Autodesk Inventor part; units mm, degrees
(part 2 of 2)
  spline S84 degree 3 poles (-140.8814, 47.3494) (-140.881, 47.3593) (-140.8802, 47.3795) (-140.879, 47.3997) (-140.8784, 47.4099) knots 0 0 0 0 0.002981 0.006062 0.006062 0.006062 0.006062 projected
  line L286 (-140.8784, 47.4099) -> (-141.648, 47.4099) projected
  spline S85 degree 3 poles (-141.648, 47.4099) (-141.7169, 47.4116) (-141.8249, 47.4142) (-141.923, 47.3709) (-141.9585, 47.3552) knots 0 0 0 0 0.02031 0.031854 0.031854 0.031854 0.031854 projected
  spline S86 degree 3 poles (-141.9585, 47.3552) (-141.9835, 47.3257) (-142.0377, 47.2619) (-142.0421, 47.1778) (-142.0445, 47.1326) knots 0 0 0 0 0.011297 0.024461 0.024461 0.024461 0.024461 projected
  line L287 (-142.0445, 47.1326) -> (-142.0445, 47.0291) projected
  line L288 (-142.0445, 47.0291) -> (-142.1167, 47.0291) projected
  line L289 (-142.1167, 47.0291) -> (-142.1167, 48.1638) projected
  line L290 (-142.1167, 48.1638) -> (-142.0445, 48.1638) projected
  line L291 (-142.0445, 48.1638) -> (-142.0445, 48.0642) projected
  spline S87 degree 3 poles (-142.0445, 48.0642) (-142.0414, 48.0133) (-142.0357, 47.9185) (-141.9669, 47.8539) (-141.9351, 47.824) knots 0 0 0 0 0.014662 0.027303 0.027303 0.027303 0.027303 projected
  spline S88 degree 3 poles (-141.9351, 47.824) (-141.9013, 47.8122) (-141.8089, 47.78) (-141.7105, 47.7818) (-141.648, 47.783) knots 0 0 0 0 0.010659 0.029193 0.029193 0.029193 0.029193 projected
  line L292 (-141.648, 47.783) -> (-139.937, 47.783) projected
  spline S89 degree 3 poles (-139.937, 47.783) (-139.8681, 47.7813) (-139.7601, 47.7787) (-139.662, 47.822) (-139.6265, 47.8377) knots 0 0 0 0 0.02031 0.031854 0.031854 0.031854 0.031854 projected
  spline S90 degree 3 poles (-139.6265, 47.8377) (-139.6015, 47.8678) (-139.5473, 47.9331) (-139.5429, 48.0184) (-139.5405, 48.0642) knots 0 0 0 0 0.011457 0.024815 0.024815 0.024815 0.024815 projected
  line L293 (-139.5405, 48.0642) -> (-139.5405, 48.1638) projected
  line L294 (-139.5405, 48.1638) -> (-139.4683, 48.1638) projected
  line L295 (-139.4683, 48.1638) -> (-139.4683, 47.199) projected
  spline S91 degree 3 poles (-139.4683, 47.199) (-139.4686, 47.0763) (-139.469, 46.8667) (-139.512, 46.6618) (-139.5298, 46.5769) knots 0 0 0 0 0.036678 0.062652 0.062652 0.062652 0.062652 projected
  spline S92 degree 3 poles (-139.5298, 46.5769) (-139.5549, 46.5125) (-139.6054, 46.3826) (-139.7058, 46.2859) (-139.7564, 46.2371) knots 0 0 0 0 0.020466 0.04128 0.04128 0.04128 0.04128 projected
  spline S93 degree 3 poles (-139.7564, 46.2371) (-139.8146, 46.1963) (-139.9328, 46.1136) (-140.0768, 46.1029) (-140.1499, 46.0974) knots 0 0 0 0 0.020904 0.042453 0.042453 0.042453 0.042453 projected
  spline S94 degree 3 poles (-140.1499, 46.0974) (-140.2285, 46.1039) (-140.3849, 46.1169) (-140.511, 46.2102) (-140.5738, 46.2566) knots 0 0 0 0 0.023147 0.04608 0.04608 0.04608 0.04608 projected
  spline S95 degree 3 poles (-140.5738, 46.2566) (-140.6301, 46.3214) (-140.7547, 46.4645) (-140.8018, 46.6489) (-140.8277, 46.7498) knots 0 0 0 0 0.02543 0.056151 0.056151 0.056151 0.056151 projected
  line L296 (-140.8277, 46.7498) -> (-141.5874, 46.2029) projected
  spline S96 degree 3 poles (-141.5874, 46.2029) (-141.6633, 46.1482) (-141.7928, 46.055) (-141.8934, 45.9317) (-141.9351, 45.8806) knots 0 0 0 0 0.027895 0.047582 0.047582 0.047582 0.047582 projected
  spline S97 degree 3 poles (-141.9351, 45.8806) (-141.9614, 45.8298) (-142.0185, 45.7192) (-142.0353, 45.5957) (-142.0445, 45.5291) knots 0 0 0 0 0.017045 0.037059 0.037059 0.037059 0.037059 projected
  line L297 (-142.0445, 45.5291) -> (-142.1167, 45.5291) projected
  circle A54 centre (-140.23, -52.19) radius 0.7 projected
  circle A55 centre (-140.23, -11.13) radius 0.7 projected
  circle A56 centre (-140.23, -6.05) radius 0.7 projected
  circle A57 centre (-140.23, -0.97) radius 0.7 projected
  circle A58 centre (-140.23, 4.11) radius 0.7 projected
  circle A59 centre (-140.23, 9.19) radius 0.7 projected
  circle A60 centre (-140.23, 11.73) radius 0.7 projected
  circle A61 centre (-140.23, 6.65) radius 0.7 projected
  circle A62 centre (-140.23, 1.57) radius 0.7 projected
  circle A63 centre (-140.23, -3.51) radius 0.7 projected
  circle A64 centre (-140.23, -8.59) radius 0.7 projected
  circle A65 centre (-140.23, -49.65) radius 0.7 projected
  circle A66 centre (-140.23, -54.73) radius 0.7 projected
  circle A67 centre (-100.1, -55.5) radius 0.7 projected
  circle A68 centre (-100.1, -45.5) radius 0.7 projected
  circle A69 centre (-100.1, -35.5) radius 0.7 projected
  circle A70 centre (-100.1, -23.5) radius 0.7 projected
  circle A71 centre (-100.1, -13.5) radius 0.7 projected
  circle A72 centre (-100.1, -3.5) radius 0.7 projected
  circle A73 centre (-100.1, 8.5) radius 0.7 projected
  circle A74 centre (-100.1, 13.5) radius 0.7 projected
  circle A75 centre (-100.1, 28.5) radius 0.7 projected
  circle A76 centre (-100.1, 40.5) radius 0.7 projected
  circle A77 centre (-100.1, 50.5) radius 0.7 projected
  circle A78 centre (-100.1, 60.5) radius 0.7 projected
  circle A79 centre (-100.1, 55.5) radius 0.7 projected
  circle A80 centre (-100.1, 45.5) radius 0.7 projected
  circle A81 centre (-100.1, 35.5) radius 0.7 projected
  circle A82 centre (-100.1, 23.5) radius 0.7 projected
  circle A83 centre (-100.1, 18.5) radius 0.7 projected
  circle A84 centre (-100.1, 3.5) radius 0.7 projected
  circle A85 centre (-100.1, -8.5) radius 0.7 projected
  circle A86 centre (-100.1, -18.5) radius 0.7 projected
  circle A87 centre (-100.1, -28.5) radius 0.7 projected
  circle A88 centre (-100.1, -40.5) radius 0.7 projected
  circle A89 centre (-100.1, -50.5) radius 0.7 projected
  circle A90 centre (-100.1, -60.5) radius 0.7 projected
  circle A91 centre (-123.2, -58) radius 0.7 projected
  circle A92 centre (-108.8682, -64) radius 0.7 projected
  circle A93 centre (-121.2, -47.4571) radius 0.7 projected
  circle A94 centre (-121.2, -35.4571) radius 0.7 projected
  circle A95 centre (-108.8682, -35.4571) radius 0.7 projected
  circle A96 centre (-123.2, -24.9143) radius 0.7 projected
  circle A97 centre (-108.8682, -30.9143) radius 0.7 projected
  circle A98 centre (-121.2, -14.3714) radius 0.7 projected
  circle A99 centre (-121.2, -2.3714) radius 0.7 projected
  circle A100 centre (-108.8682, -2.3714) radius 0.7 projected
  circle A101 centre (-123.2, 8.1714) radius 0.7 projected
  circle A102 centre (-108.8682, 2.1714) radius 0.7 projected
  circle A103 centre (-121.2, 18.7143) radius 0.7 projected
  circle A104 centre (-121.2, 30.7143) radius 0.7 projected
  circle A105 centre (-108.8682, 30.7143) radius 0.7 projected
  circle A106 centre (-123.2, 41.2571) radius 0.7 projected
  circle A107 centre (-108.8682, 35.2571) radius 0.7 projected
  circle A108 centre (-121.2, 51.8) radius 0.7 projected
  circle A109 centre (-121.2, 63.8) radius 0.7 projected
  circle A110 centre (-108.8682, 63.8) radius 0.7 projected
  circle A111 centre (-108.8682, 51.8) radius 0.7 projected
  circle A112 centre (-123.2, 57.8) radius 0.7 projected
  circle A113 centre (-108.8682, 47.2571) radius 0.7 projected
  circle A114 centre (-121.2, 47.2571) radius 0.7 projected
  circle A115 centre (-121.2, 35.2571) radius 0.7 projected
  circle A116 centre (-108.8682, 18.7143) radius 0.7 projected
  circle A117 centre (-123.2, 24.7143) radius 0.7 projected
  circle A118 centre (-108.8682, 14.1714) radius 0.7 projected
  circle A119 centre (-121.2, 14.1714) radius 0.7 projected
  circle A120 centre (-121.2, 2.1714) radius 0.7 projected
  circle A121 centre (-108.8682, -14.3714) radius 0.7 projected
  circle A122 centre (-123.2, -8.3714) radius 0.7 projected
  circle A123 centre (-108.8682, -18.9143) radius 0.7 projected
  circle A124 centre (-121.2, -18.9143) radius 0.7 projected
  circle A125 centre (-121.2, -30.9143) radius 0.7 projected
  circle A126 centre (-108.8682, -47.4571) radius 0.7 projected
  circle A127 centre (-123.2, -41.4571) radius 0.7 projected
  circle A128 centre (-108.8682, -52) radius 0.7 projected
  circle A129 centre (-121.2, -52) radius 0.7 projected
  circle A130 centre (-121.2, -64) radius 0.7 projected
  circle A131 centre (-97, -66) radius 1.55 projected
  circle A132 centre (-141, -66) radius 1.55 projected
  circle A133 centre (-141, 66) radius 1.55 projected
  circle A134 centre (-97, 66) radius 1.55 projected
  line L298 (-139.3394, 43.0486) -> (-141.7124, 43.0486) projected
  spline S98 degree 3 poles (-141.7124, 43.0486) (-141.7593, 43.049) (-141.8347, 43.0498) (-141.9075, 43.0312) (-141.9351, 43.0242) knots 0 0 0 0 0.013978 0.022479 0.022479 0.022479 0.022479 projected
  spline S99 degree 3 poles (-141.9351, 43.0242) (-141.9522, 43.015) (-141.9861, 42.9968) (-142.0075, 42.9648) (-142.0181, 42.949) knots 0 0 0 0 0.005722 0.011354 0.011354 0.011354 0.011354 projected
  spline S100 degree 3 poles (-142.0181, 42.949) (-142.0263, 42.9249) (-142.047, 42.8637) (-142.0466, 42.7989) (-142.0464, 42.7595) knots 0 0 0 0 0.007579 0.019271 0.019271 0.019271 0.019271 projected
  line L299 (-142.0464, 42.7595) -> (-142.1167, 42.7595) projected
  line L300 (-142.1167, 42.7595) -> (-142.1167, 43.6365) projected
  line L301 (-142.1167, 43.6365) -> (-142.0464, 43.6365) projected
  spline S101 degree 3 poles (-142.0464, 43.6365) (-142.0466, 43.6016) (-142.047, 43.544) (-142.0283, 43.4898) (-142.021, 43.4685) knots 0 0 0 0 0.010371 0.017092 0.017092 0.017092 0.017092 projected
  spline S102 degree 3 poles (-142.021, 43.4685) (-142.0107, 43.4541) (-141.9887, 43.4237) (-141.9549, 43.407) (-141.937, 43.3982) knots 0 0 0 0 0.005233 0.011103 0.011103 0.011103 0.011103 projected
  spline S103 degree 3 poles (-141.937, 43.3982) (-141.9087, 43.3909) (-141.8352, 43.3719) (-141.7591, 43.3725) (-141.7124, 43.3728) knots 0 0 0 0 0.008755 0.022685 0.022685 0.022685 0.022685 projected
  line L302 (-141.7124, 43.3728) -> (-140.0874, 43.3728) projected
  spline S104 degree 3 poles (-140.0874, 43.3728) (-140.0059, 43.3722) (-139.8816, 43.3712) (-139.7579, 43.3826) (-139.7154, 43.3865) knots 0 0 0 0 0.024441 0.037251 0.037251 0.037251 0.037251 projected
  spline S105 degree 3 poles (-139.7154, 43.3865) (-139.6951, 43.3907) (-139.6599, 43.3981) (-139.6323, 43.4208) (-139.6206, 43.4304) knots 0 0 0 0 0.006101 0.01058 0.01058 0.01058 0.01058 projected
  spline S106 degree 3 poles (-139.6206, 43.4304) (-139.6132, 43.4415) (-139.5977, 43.4649) (-139.5961, 43.4929) (-139.5952, 43.5076) knots 0 0 0 0 0.003934 0.008253 0.008253 0.008253 0.008253 projected
  spline S107 degree 3 poles (-139.5952, 43.5076) (-139.5971, 43.527) (-139.6013, 43.5713) (-139.6174, 43.613) (-139.6265, 43.6365) knots 0 0 0 0 0.005814 0.013319 0.013319 0.013319 0.013319 projected
  line L303 (-139.6265, 43.6365) -> (-139.5581, 43.6697) projected
  line L304 (-139.5581, 43.6697) -> (-139.3394, 43.1365) projected
  line L305 (-139.3394, 43.1365) -> (-139.3394, 43.0486) projected
  line L306 (-140.3277, 40.8787) -> (-140.3277, 40.0447) projected
  line L307 (-140.3277, 40.0447) -> (-140.3999, 40.0447) projected
  line L308 (-140.3999, 40.0447) -> (-140.3999, 40.0857) projected
  spline S108 degree 3 poles (-140.3999, 40.0857) (-140.4007, 40.1121) (-140.402, 40.1596) (-140.4269, 40.1997) (-140.438, 40.2175) knots 0 0 0 0 0.007749 0.013941 0.013941 0.013941 0.013941 projected
  spline S109 degree 3 poles (-140.438, 40.2175) (-140.4514, 40.2304) (-140.478, 40.2558) (-140.5146, 40.2596) (-140.5327, 40.2615) knots 0 0 0 0 0.005396 0.010711 0.010711 0.010711 0.010711 projected
  spline S110 degree 3 poles (-140.5327, 40.2615) (-140.5634, 40.2574) (-140.637, 40.2475) (-140.7044, 40.2156) (-140.7437, 40.197) knots 0 0 0 0 0.009224 0.022172 0.022172 0.022172 0.022172 projected
  line L309 (-140.7437, 40.197) -> (-141.646, 39.7615) projected
  line L310 (-141.646, 39.7615) -> (-140.6577, 39.3611) projected
  spline S111 degree 3 poles (-140.6577, 39.3611) (-140.6315, 39.3514) (-140.5804, 39.3325) (-140.526, 39.3294) (-140.4995, 39.3279) knots 0 0 0 0 0.008339 0.016245 0.016245 0.016245 0.016245 projected
  spline S112 degree 3 poles (-140.4995, 39.3279) (-140.489, 39.3281) (-140.4703, 39.3285) (-140.454, 39.3376) (-140.4468, 39.3416) knots 0 0 0 0 0.003095 0.00552 0.00552 0.00552 0.00552 projected
  spline S113 degree 3 poles (-140.4468, 39.3416) (-140.4399, 39.3479) (-140.4249, 39.3616) (-140.4169, 39.3803) (-140.4126, 39.3904) knots 0 0 0 0 0.00278 0.006023 0.006023 0.006023 0.006023 projected
  spline S114 degree 3 poles (-140.4126, 39.3904) (-140.409, 39.4056) (-140.3997, 39.4441) (-140.3998, 39.4837) (-140.3999, 39.5076) knots 0 0 0 0 0.004688 0.011824 0.011824 0.011824 0.011824 projected
  line L311 (-140.3999, 39.5076) -> (-140.3277, 39.5076) projected
  line L312 (-140.3277, 39.5076) -> (-140.3277, 38.9255) projected
  line L313 (-140.3277, 38.9255) -> (-140.3999, 38.9255) projected
  spline S115 degree 3 poles (-140.3999, 38.9255) (-140.4026, 38.9472) (-140.4074, 38.986) (-140.4239, 39.0213) (-140.4312, 39.0369) knots 0 0 0 0 0.006503 0.011626 0.011626 0.011626 0.011626 projected
  spline S116 degree 3 poles (-140.4312, 39.0369) (-140.4419, 39.0511) (-140.4668, 39.0841) (-140.5001, 39.1087) (-140.5191, 39.1228) knots 0 0 0 0 0.005308 0.012347 0.012347 0.012347 0.012347 projected
  spline S117 degree 3 poles (-140.5191, 39.1228) (-140.5361, 39.1315) (-140.5849, 39.1564) (-140.6361, 39.1763) (-140.6695, 39.1892) knots 0 0 0 0 0.005721 0.016448 0.016448 0.016448 0.016448 projected
  line L314 (-140.6695, 39.1892) -> (-142.4546, 39.9177) projected
  spline S118 degree 3 poles (-142.4546, 39.9177) (-142.5341, 39.9534) (-142.6831, 40.0203) (-142.795, 40.1388) (-142.8472, 40.1941) knots 0 0 0 0 0.025853 0.048427 0.048427 0.048427 0.048427 projected
  spline S119 degree 3 poles (-142.8472, 40.1941) (-142.8858, 40.2479) (-142.9571, 40.3471) (-142.9728, 40.4679) (-142.98, 40.5232) knots 0 0 0 0 0.019507 0.035983 0.035983 0.035983 0.035983 projected
  spline S120 degree 3 poles (-142.98, 40.5232) (-142.9777, 40.5594) (-142.9733, 40.6289) (-142.933, 40.6855) (-142.9136, 40.7127) knots 0 0 0 0 0.010629 0.020435 0.020435 0.020435 0.020435 projected
  spline S121 degree 3 poles (-142.9136, 40.7127) (-142.8913, 40.7343) (-142.8485, 40.7758) (-142.7895, 40.7833) (-142.7613, 40.7869) knots 0 0 0 0 0.009045 0.01736 0.01736 0.01736 0.01736 projected
  spline S122 degree 3 poles (-142.7613, 40.7869) (-142.7355, 40.7849) (-142.6857, 40.7812) (-142.6478, 40.7488) (-142.6294, 40.7332) knots 0 0 0 0 0.007518 0.014569 0.014569 0.014569 0.014569 projected
  spline S123 degree 3 poles (-142.6294, 40.7332) (-142.6149, 40.7126) (-142.5838, 40.6686) (-142.5811, 40.6146) (-142.5796, 40.5857) knots 0 0 0 0 0.007386 0.015852 0.015852 0.015852 0.015852 projected
  spline S124 degree 3 poles (-142.5796, 40.5857) (-142.5823, 40.5601) (-142.5886, 40.4997) (-142.6101, 40.4427) (-142.6226, 40.4099) knots 0 0 0 0 0.007693 0.018162 0.018162 0.018162 0.018162 projected
  spline S125 degree 3 poles (-142.6226, 40.4099) (-142.6308, 40.389) (-142.6432, 40.3572) (-142.6497, 40.3237) (-142.6519, 40.3123) knots 0 0 0 0 0.006717 0.010213 0.010213 0.010213 0.010213 projected
  spline S126 degree 3 poles (-142.6519, 40.3123) (-142.6483, 40.2912) (-142.6402, 40.2431) (-142.6089, 40.2055) (-142.5913, 40.1843) knots 0 0 0 0 0.006312 0.014377 0.014377 0.014377 0.014377 projected
  spline S127 degree 3 poles (-142.5913, 40.1843) (-142.5626, 40.1597) (-142.4927, 40.0999) (-142.4073, 40.0651) (-142.357, 40.0447) knots 0 0 0 0 0.011287 0.027437 0.027437 0.027437 0.027437 projected
  line L315 (-142.357, 40.0447) -> (-142.0464, 39.9177) projected
  line L316 (-142.0464, 39.9177) -> (-140.6968, 40.5603) projected
  spline S128 degree 3 poles (-140.6968, 40.5603) (-140.6739, 40.5726) (-140.6218, 40.6006) (-140.5735, 40.6349) (-140.5464, 40.6541) knots 0 0 0 0 0.007783 0.017737 0.017737 0.017737 0.017737 projected
  spline S129 degree 3 poles (-140.5464, 40.6541) (-140.5267, 40.6681) (-140.4935, 40.6919) (-140.4659, 40.7219) (-140.4546, 40.7341) knots 0 0 0 0 0.007237 0.01221 0.01221 0.01221 0.01221 projected
  spline S130 degree 3 poles (-140.4546, 40.7341) (-140.4441, 40.7534) (-140.4192, 40.7989) (-140.407, 40.8495) (-140.3999, 40.8787) knots 0 0 0 0 0.006551 0.015512 0.015512 0.015512 0.015512 projected
  line L317 (-140.3999, 40.8787) -> (-140.3277, 40.8787) projected
  line L318 (-142.1167, 36.2654) -> (-139.8882, 37.2888) projected
  line L319 (-139.8882, 37.2888) -> (-141.6577, 37.2888) projected
  spline S131 degree 3 poles (-141.6577, 37.2888) (-141.7251, 37.2904) (-141.8309, 37.2928) (-141.9274, 37.2512) (-141.9624, 37.2361) knots 0 0 0 0 0.019868 0.031224 0.031224 0.031224 0.031224 projected
  spline S132 degree 3 poles (-141.9624, 37.2361) (-141.9863, 37.2063) (-142.0394, 37.14) (-142.0426, 37.0546) (-142.0445, 37.0076) knots 0 0 0 0 0.011173 0.024853 0.024853 0.024853 0.024853 projected
  line L320 (-142.0445, 37.0076) -> (-142.0445, 36.9138) projected
  line L321 (-142.0445, 36.9138) -> (-142.1167, 36.9138) projected
  line L322 (-142.1167, 36.9138) -> (-142.1167, 37.8357) projected
  line L323 (-142.1167, 37.8357) -> (-142.0445, 37.8357) projected
  line L324 (-142.0445, 37.8357) -> (-142.0445, 37.742) projected
  spline S133 degree 3 poles (-142.0445, 37.742) (-142.042, 37.6914) (-142.0375, 37.5986) (-141.9724, 37.5334) (-141.9429, 37.5037) knots 0 0 0 0 0.014578 0.026734 0.026734 0.026734 0.026734 projected
  spline S134 degree 3 poles (-141.9429, 37.5037) (-141.909, 37.4913) (-141.8174, 37.458) (-141.7195, 37.4597) (-141.6577, 37.4607) knots 0 0 0 0 0.010748 0.029042 0.029042 0.029042 0.029042 projected
  line L325 (-141.6577, 37.4607) -> (-139.9273, 37.4607) projected
  spline S135 degree 3 poles (-139.9273, 37.4607) (-139.8763, 37.4608) (-139.7894, 37.4611) (-139.7073, 37.4885) (-139.6734, 37.4998) knots 0 0 0 0 0.015168 0.025832 0.025832 0.025832 0.025832 projected
  spline S136 degree 3 poles (-139.6734, 37.4998) (-139.6549, 37.5116) (-139.615, 37.5371) (-139.5913, 37.5783) (-139.5786, 37.6004) knots 0 0 0 0 0.006489 0.014 0.014 0.014 0.014 projected
  spline S137 degree 3 poles (-139.5786, 37.6004) (-139.5676, 37.6319) (-139.541, 37.7078) (-139.5407, 37.7885) (-139.5405, 37.8357) knots 0 0 0 0 0.009964 0.023986 0.023986 0.023986 0.023986 projected
  line L326 (-139.5405, 37.8357) -> (-139.4683, 37.8357) projected
  line L327 (-139.4683, 37.8357) -> (-139.4683, 37.0857) projected
  line L328 (-139.4683, 37.0857) -> (-141.5405, 36.1248) projected
  line L329 (-141.5405, 36.1248) -> (-139.4683, 35.1795) projected
  line L330 (-139.4683, 35.1795) -> (-139.4683, 34.4295) projected
  line L331 (-139.4683, 34.4295) -> (-139.5405, 34.4295) projected
  line L332 (-139.5405, 34.4295) -> (-139.5405, 34.5212) projected
  spline S138 degree 3 poles (-139.5405, 34.5212) (-139.5429, 34.5723) (-139.5473, 34.6657) (-139.6126, 34.7316) (-139.6421, 34.7615) knots 0 0 0 0 0.014723 0.026916 0.026916 0.026916 0.026916 projected
  spline S139 degree 3 poles (-139.6421, 34.7615) (-139.676, 34.7738) (-139.7676, 34.8072) (-139.8655, 34.8055) (-139.9273, 34.8045) knots 0 0 0 0 0.010748 0.029042 0.029042 0.029042 0.029042 projected
  line L333 (-139.9273, 34.8045) -> (-141.6577, 34.8045) projected
  spline S140 degree 3 poles (-141.6577, 34.8045) (-141.7252, 34.806) (-141.8313, 34.8085) (-141.9274, 34.7655) (-141.9624, 34.7498) knots 0 0 0 0 0.019871 0.031279 0.031279 0.031279 0.031279 projected
  spline S141 degree 3 poles (-141.9624, 34.7498) (-141.9863, 34.72) (-142.0394, 34.6537) (-142.0426, 34.5683) (-142.0445, 34.5212) knots 0 0 0 0 0.011173 0.024853 0.024853 0.024853 0.024853 projected
  line L334 (-142.0445, 34.5212) -> (-142.0445, 34.4295) projected
  line L335 (-142.0445, 34.4295) -> (-142.1167, 34.4295) projected
  line L336 (-142.1167, 34.4295) -> (-142.1167, 35.5545) projected
  line L337 (-142.1167, 35.5545) -> (-142.0445, 35.5545) projected
  line L338 (-142.0445, 35.5545) -> (-142.0445, 35.4607) projected
  spline S142 degree 3 poles (-142.0445, 35.4607) (-142.0421, 35.4097) (-142.0379, 35.3168) (-141.9724, 35.2518) (-141.9429, 35.2224) knots 0 0 0 0 0.014674 0.026754 0.026754 0.026754 0.026754 projected
  spline S143 degree 3 poles (-141.9429, 35.2224) (-141.909, 35.2101) (-141.8174, 35.1767) (-141.7195, 35.1784) (-141.6577, 35.1795) knots 0 0 0 0 0.010748 0.029042 0.029042 0.029042 0.029042 projected
  line L339 (-141.6577, 35.1795) -> (-139.8882, 35.1795) projected
  line L340 (-139.8882, 35.1795) -> (-142.1167, 36.2009) projected
  line L341 (-142.1167, 36.2009) -> (-142.1167, 36.2654) projected
  spline S144 degree 3 poles (-141.9155, 30.9568) (-141.9569, 30.9982) (-142.0336, 31.075) (-142.0872, 31.1693) (-142.1118, 31.2127) knots 0 0 0 0 0.017474 0.032377 0.032377 0.032377 0.032377 projected
  spline S145 degree 3 poles (-142.1118, 31.2127) (-142.1292, 31.2554) (-142.1643, 31.3418) (-142.169, 31.4351) (-142.1714, 31.4822) knots 0 0 0 0 0.013735 0.027779 0.027779 0.027779 0.027779 projected
  spline S146 degree 3 poles (-142.1714, 31.4822) (-142.1599, 31.5779) (-142.1362, 31.7757) (-141.9978, 31.9196) (-141.9263, 31.9939) knots 0 0 0 0 0.028117 0.058136 0.058136 0.058136 0.058136 projected
  spline S147 degree 3 poles (-141.9263, 31.9939) (-141.8362, 32.0577) (-141.6478, 32.191) (-141.4169, 32.2052) (-141.2964, 32.2127) knots 0 0 0 0 0.032455 0.067865 0.067865 0.067865 0.067865 projected
  spline S148 degree 3 poles (-141.2964, 32.2127) (-141.1703, 32.2021) (-140.9153, 32.1808) (-140.7008, 32.0411) (-140.5923, 31.9705) knots 0 0 0 0 0.037335 0.075504 0.075504 0.075504 0.075504 projected
  spline S149 degree 3 poles (-140.5923, 31.9705) (-140.4992, 31.8849) (-140.3157, 31.7164) (-140.2871, 31.4692) (-140.273, 31.3474) knots 0 0 0 0 0.036607 0.072135 0.072135 0.072135 0.072135 projected
  spline S150 degree 3 poles (-140.273, 31.3474) (-140.2786, 31.2728) (-140.2895, 31.1272) (-140.3795, 31.0126) (-140.4234, 30.9568) knots 0 0 0 0 0.021907 0.042711 0.042711 0.042711 0.042711 projected
  line L342 (-140.4234, 30.9568) -> (-140.0933, 30.9568) projected
  spline S151 degree 3 poles (-140.0933, 30.9568) (-140.0107, 30.9561) (-139.8847, 30.9551) (-139.7594, 30.9673) (-139.7163, 30.9714) knots 0 0 0 0 0.024759 0.037745 0.037745 0.037745 0.037745 projected
  spline S152 degree 3 poles (-139.7163, 30.9714) (-139.6957, 30.976) (-139.66, 30.9838) (-139.6324, 31.0074) (-139.6206, 31.0173) knots 0 0 0 0 0.0062 0.010756 0.010756 0.010756 0.010756 projected
  spline S153 degree 3 poles (-139.6206, 31.0173) (-139.6132, 31.0287) (-139.5978, 31.0524) (-139.5961, 31.0807) (-139.5952, 31.0955) knots 0 0 0 0 0.003998 0.008342 0.008342 0.008342 0.008342 projected
  spline S154 degree 3 poles (-139.5952, 31.0955) (-139.5971, 31.1153) (-139.6016, 31.1616) (-139.6174, 31.2053) (-139.6265, 31.2302) knots 0 0 0 0 0.00596 0.013883 0.013883 0.013883 0.013883 projected
  line L343 (-139.6265, 31.2302) -> (-139.5581, 31.2556) projected
  line L344 (-139.5581, 31.2556) -> (-139.3394, 30.7224) projected
  line L345 (-139.3394, 30.7224) -> (-139.3394, 30.6345) projected
  line L346 (-139.3394, 30.6345) -> (-141.4077, 30.6345) projected
  spline S155 degree 3 poles (-141.4077, 30.6345) (-141.4922, 30.6352) (-141.6204, 30.6363) (-141.748, 30.6241) (-141.7915, 30.6199) knots 0 0 0 0 0.02532 0.038428 0.038428 0.038428 0.038428 projected
  spline S156 degree 3 poles (-141.7915, 30.6199) (-141.812, 30.6152) (-141.848, 30.607) (-141.8761, 30.5832) (-141.8882, 30.573) knots 0 0 0 0 0.006184 0.010882 0.010882 0.010882 0.010882 projected
  spline S157 degree 3 poles (-141.8882, 30.573) (-141.8962, 30.5618) (-141.9122, 30.5392) (-141.9144, 30.5117) (-141.9155, 30.4978) knots 0 0 0 0 0.004049 0.008135 0.008135 0.008135 0.008135 projected
  spline S158 degree 3 poles (-141.9155, 30.4978) (-141.9135, 30.4771) (-141.9088, 30.4289) (-141.892, 30.3833) (-141.8823, 30.3572) knots 0 0 0 0 0.006208 0.014501 0.014501 0.014501 0.014501 projected
  line L347 (-141.8823, 30.3572) -> (-141.9507, 30.3357) projected
  line L348 (-141.9507, 30.3357) -> (-142.1714, 30.867) projected
  line L349 (-142.1714, 30.867) -> (-142.1714, 30.9568) projected
  line L350 (-142.1714, 30.9568) -> (-141.9155, 30.9568) projected
  spline S159 degree 3 poles (-141.0015, 26.8084) (-141.1236, 26.8037) (-141.35, 26.795) (-141.5393, 26.6718) (-141.6265, 26.615) knots 0 0 0 0 0.035861 0.066514 0.066514 0.066514 0.066514 projected
  spline S160 degree 3 poles (-141.6265, 26.615) (-141.6925, 26.5487) (-141.82, 26.4209) (-141.8423, 26.2421) (-141.853, 26.156) knots 0 0 0 0 0.027201 0.052501 0.052501 0.052501 0.052501 projected
  spline S161 degree 3 poles (-141.853, 26.156) (-141.8494, 26.0998) (-141.8422, 25.9899) (-141.7846, 25.8962) (-141.7564, 25.8504) knots 0 0 0 0 0.016607 0.032494 0.032494 0.032494 0.032494 projected
  spline S162 degree 3 poles (-141.7564, 25.8504) (-141.7147, 25.8075) (-141.6208, 25.7109) (-141.4952, 25.6606) (-141.4253, 25.6326) knots 0 0 0 0 0.017732 0.040016 0.040016 0.040016 0.040016 projected
  line L351 (-141.4253, 25.6326) -> (-141.4644, 25.572) projected
  spline S163 degree 3 poles (-141.4644, 25.572) (-141.5524, 25.5929) (-141.7326, 25.6358) (-141.8775, 25.7512) (-141.9517, 25.8103) knots 0 0 0 0 0.026786 0.054841 0.054841 0.054841 0.054841 projected
  spline S164 degree 3 poles (-141.9517, 25.8103) (-142.0158, 25.8803) (-142.1441, 26.0205) (-142.1623, 26.2097) (-142.1714, 26.3045) knots 0 0 0 0 0.027662 0.055408 0.055408 0.055408 0.055408 projected
  spline S165 degree 3 poles (-142.1714, 26.3045) (-142.1603, 26.4086) (-142.1378, 26.6201) (-141.9936, 26.7767) (-141.9204, 26.8562) knots 0 0 0 0 0.030558 0.062067 0.062067 0.062067 0.062067 projected
  spline S166 degree 3 poles (-141.9204, 26.8562) (-141.8257, 26.9231) (-141.6241, 27.0655) (-141.3768, 27.0787) (-141.2456, 27.0857) knots 0 0 0 0 0.034084 0.072576 0.072576 0.072576 0.072576 projected
  spline S167 degree 3 poles (-141.2456, 27.0857) (-141.1049, 27.0792) (-140.8434, 27.0672) (-140.6289, 26.9189) (-140.5298, 26.8503) knots 0 0 0 0 0.041266 0.076711 0.076711 0.076711 0.076711 projected
  spline S168 degree 3 poles (-140.5298, 26.8503) (-140.4549, 26.7666) (-140.3042, 26.598) (-140.2834, 26.3728) (-140.273, 26.2595) knots 0 0 0 0 0.032792 0.065963 0.065963 0.065963 0.065963 projected
  spline S169 degree 3 poles (-140.273, 26.2595) (-140.2804, 26.1645) (-140.295, 25.9789) (-140.4134, 25.8354) (-140.4712, 25.7654) knots 0 0 0 0 0.027837 0.054408 0.054408 0.054408 0.054408 projected
  spline S170 degree 3 poles (-140.4712, 25.7654) (-140.5454, 25.709) (-140.7018, 25.5903) (-140.8983, 25.5783) (-141.0015, 25.572) knots 0 0 0 0 0.027333 0.05758 0.05758 0.05758 0.05758 projected
  line L352 (-141.0015, 25.572) -> (-141.0015, 26.8084) projected
  spline S171 degree 3 poles (-141.0015, 45.1384) (-141.1236, 45.1337) (-141.35, 45.125) (-141.5393, 45.0018) (-141.6265, 44.9451) knots 0 0 0 0 0.035861 0.066514 0.066514 0.066514 0.066514 projected
  spline S172 degree 3 poles (-141.6265, 44.9451) (-141.6925, 44.8788) (-141.82, 44.751) (-141.8423, 44.5722) (-141.853, 44.4861) knots 0 0 0 0 0.027201 0.052501 0.052501 0.052501 0.052501 projected
  spline S173 degree 3 poles (-141.853, 44.4861) (-141.8494, 44.4299) (-141.8422, 44.32) (-141.7846, 44.2263) (-141.7564, 44.1804) knots 0 0 0 0 0.016607 0.032494 0.032494 0.032494 0.032494 projected
  spline S174 degree 3 poles (-141.7564, 44.1804) (-141.7147, 44.1376) (-141.6208, 44.0409) (-141.4952, 43.9907) (-141.4253, 43.9627) knots 0 0 0 0 0.017732 0.040016 0.040016 0.040016 0.040016 projected
  line L353 (-141.4253, 43.9627) -> (-141.4644, 43.9021) projected
  spline S175 degree 3 poles (-141.4644, 43.9021) (-141.5524, 43.923) (-141.7326, 43.9658) (-141.8775, 44.0813) (-141.9517, 44.1404) knots 0 0 0 0 0.026786 0.054841 0.054841 0.054841 0.054841 projected
  spline S176 degree 3 poles (-141.9517, 44.1404) (-142.0158, 44.2104) (-142.1441, 44.3505) (-142.1623, 44.5398) (-142.1714, 44.6345) knots 0 0 0 0 0.027662 0.055408 0.055408 0.055408 0.055408 projected
  spline S177 degree 3 poles (-142.1714, 44.6345) (-142.1603, 44.7387) (-142.1378, 44.9501) (-141.9936, 45.1068) (-141.9204, 45.1863) knots 0 0 0 0 0.030558 0.062067 0.062067 0.062067 0.062067 projected
  spline S178 degree 3 poles (-141.9204, 45.1863) (-141.8257, 45.2532) (-141.6241, 45.3955) (-141.3768, 45.4088) (-141.2456, 45.4158) knots 0 0 0 0 0.034084 0.072576 0.072576 0.072576 0.072576 projected
  spline S179 degree 3 poles (-141.2456, 45.4158) (-141.1049, 45.4093) (-140.8434, 45.3973) (-140.6289, 45.249) (-140.5298, 45.1804) knots 0 0 0 0 0.041266 0.076711 0.076711 0.076711 0.076711 projected
  spline S180 degree 3 poles (-140.5298, 45.1804) (-140.4549, 45.0966) (-140.3042, 44.9281) (-140.2834, 44.7029) (-140.273, 44.5896) knots 0 0 0 0 0.032792 0.065963 0.065963 0.065963 0.065963 projected
  spline S181 degree 3 poles (-140.273, 44.5896) (-140.2804, 44.4946) (-140.295, 44.3089) (-140.4134, 44.1655) (-140.4712, 44.0955) knots 0 0 0 0 0.027837 0.054408 0.054408 0.054408 0.054408 projected
  spline S182 degree 3 poles (-140.4712, 44.0955) (-140.5454, 44.0391) (-140.7018, 43.9204) (-140.8983, 43.9084) (-141.0015, 43.9021) knots 0 0 0 0 0.027333 0.05758 0.05758 0.05758 0.05758 projected
  line L354 (-141.0015, 43.9021) -> (-141.0015, 45.1384) projected
  line L355 (-127.3, -52) -> (-127.3, -53) projected
  line L356 (-127.3, -53) -> (-127.6, -53) projected
  line L357 (-127.6, -53) -> (-127.6, -52.3) projected
  line L358 (-127.6, -52.3) -> (-129.5, -52.3) projected
  line L359 (-129.5, -52.3) -> (-129.5, -52) projected
  line L360 (-129.5, -52) -> (-127.3, -52) projected
  line L361 (-135.5, -35.4571) -> (-133.2, -35.4571) projected
  line L362 (-133.2, -35.4571) -> (-133.2, -40.6571) projected
  line L363 (-133.2, -40.6571) -> (-135.5, -40.6571) projected
  line L364 (-135.5, -40.6571) -> (-135.5, -35.4571) projected
  line L365 (-128.7, -25.1143) -> (-126, -25.1143) projected
  line L366 (-126, -25.1143) -> (-126, -22.7143) projected
  line L367 (-126, -22.7143) -> (-124.2, -20.9143) projected
  line L368 (-124.2, -20.9143) -> (-119.5, -20.9143) projected
  line L369 (-119.5, -20.9143) -> (-119.5, -22.0143) projected
  line L370 (-119.5, -22.0143) -> (-123.8858, -22.0143) projected
  line L371 (-123.8858, -22.0143) -> (-124.9, -23.0285) projected
  line L372 (-124.9, -23.0285) -> (-124.9, -26.8001) projected
  line L373 (-124.9, -26.8001) -> (-123.8858, -27.8143) projected
  line L374 (-123.8858, -27.8143) -> (-119.5, -27.8143) projected
  line L375 (-119.5, -27.8143) -> (-119.5, -28.9143) projected
  line L376 (-119.5, -28.9143) -> (-124.2, -28.9143) projected
  line L377 (-124.2, -28.9143) -> (-126, -27.1143) projected
  line L378 (-126, -27.1143) -> (-126, -31.8143) projected
  line L379 (-126, -31.8143) -> (-128.7, -31.8143) projected
  line L380 (-128.7, -31.8143) -> (-128.7, -25.1143) projected
  line L381 (-128.7, -8.5714) -> (-126, -8.5714) projected
  line L382 (-126, -8.5714) -> (-126, -6.1714) projected
  line L383 (-126, -6.1714) -> (-124.2, -4.3714) projected
  line L384 (-124.2, -4.3714) -> (-119.5, -4.3714) projected
  line L385 (-119.5, -4.3714) -> (-119.5, -5.4714) projected
  line L386 (-119.5, -5.4714) -> (-123.8858, -5.4714) projected
  line L387 (-123.8858, -5.4714) -> (-124.9, -6.4856) projected
  line L388 (-124.9, -6.4856) -> (-124.9, -10.2572) projected
  line L389 (-124.9, -10.2572) -> (-123.8858, -11.2714) projected
  line L390 (-123.8858, -11.2714) -> (-119.5, -11.2714) projected
  line L391 (-119.5, -11.2714) -> (-119.5, -12.3714) projected
  line L392 (-119.5, -12.3714) -> (-124.2, -12.3714) projected
  line L393 (-124.2, -12.3714) -> (-126, -10.5714) projected
  line L394 (-126, -10.5714) -> (-126, -15.2714) projected
  line L395 (-126, -15.2714) -> (-128.7, -15.2714) projected
  line L396 (-128.7, -15.2714) -> (-128.7, -8.5714) projected
  line L397 (-135.5, -2.3714) -> (-133.2, -2.3714) projected
  line L398 (-133.2, -2.3714) -> (-133.2, -7.5714) projected
  line L399 (-133.2, -7.5714) -> (-135.5, -7.5714) projected
  line L400 (-135.5, -7.5714) -> (-135.5, -2.3714) projected
  line L401 (-127.3, 14.1714) -> (-127.3, 13.1714) projected
  line L402 (-127.3, 13.1714) -> (-127.6, 13.1714) projected
  line L403 (-127.6, 13.1714) -> (-127.6, 13.8714) projected
  line L404 (-127.6, 13.8714) -> (-129.5, 13.8714) projected
  line L405 (-129.5, 13.8714) -> (-129.5, 14.1714) projected
  line L406 (-129.5, 14.1714) -> (-127.3, 14.1714) projected
  line L407 (-137, 17.8143) -> (-137, 23.4143) projected
  line L408 (-137, 23.4143) -> (-131, 23.4143) projected
  line L409 (-131, 23.4143) -> (-131, 17.8143) projected
  line L410 (-131, 17.8143) -> (-137, 17.8143) projected
  line L411 (-133, 47.2571) -> (-130.7, 47.2571) projected
  line L412 (-130.7, 47.2571) -> (-130.7, 42.0571) projected
  line L413 (-130.7, 42.0571) -> (-133, 42.0571) projected
  line L414 (-133, 42.0571) -> (-133, 47.2571) projected
  line L415 (-135.5, 58.6) -> (-135.5, 63.8) projected
  line L416 (-135.5, 63.8) -> (-133.2, 63.8) projected
  line L417 (-133.2, 63.8) -> (-133.2, 58.6) projected
  line L418 (-133.2, 58.6) -> (-135.5, 58.6) projected
  line L419 (-127.6, 60.9) -> (-127.6, 61.6) projected
  line L420 (-127.6, 61.6) -> (-127.3, 61.6) projected
  line L421 (-127.3, 61.6) -> (-127.3, 60.6) projected
  line L422 (-127.3, 60.6) -> (-129.5, 60.6) projected
  line L423 (-129.5, 60.6) -> (-129.5, 60.9) projected
  line L424 (-129.5, 60.9) -> (-127.6, 60.9) projected
  line L425 (-127.3, 47.2571) -> (-127.3, 46.2571) projected
  line L426 (-127.3, 46.2571) -> (-127.6, 46.2571) projected
  line L427 (-127.6, 46.2571) -> (-127.6, 46.9571) projected
  line L428 (-127.6, 46.9571) -> (-129.5, 46.9571) projected
  line L429 (-129.5, 46.9571) -> (-129.5, 47.2571) projected
  line L430 (-129.5, 47.2571) -> (-127.3, 47.2571) projected
  line L431 (-127.3, 30.7143) -> (-127.3, 29.7143) projected
  line L432 (-127.3, 29.7143) -> (-127.6, 29.7143) projected
  line L433 (-127.6, 29.7143) -> (-127.6, 30.4143) projected
  line L434 (-127.6, 30.4143) -> (-129.5, 30.4143) projected
  line L435 (-129.5, 30.4143) -> (-129.5, 30.7143) projected
  line L436 (-129.5, 30.7143) -> (-127.3, 30.7143) projected
  line L437 (-133, 30.7143) -> (-130.7, 30.7143) projected
  line L438 (-130.7, 30.7143) -> (-130.7, 25.5143) projected
  line L439 (-130.7, 25.5143) -> (-133, 25.5143) projected
  line L440 (-133, 25.5143) -> (-133, 30.7143) projected
  line L441 (-133, -2.3714) -> (-130.7, -2.3714) projected
  line L442 (-130.7, -2.3714) -> (-130.7, -7.5714) projected
  line L443 (-130.7, -7.5714) -> (-133, -7.5714) projected
  line L444 (-133, -7.5714) -> (-133, -2.3714) projected
  line L445 (-133, -18.9143) -> (-130.7, -18.9143) projected
  line L446 (-130.7, -18.9143) -> (-130.7, -24.1143) projected
  line L447 (-130.7, -24.1143) -> (-133, -24.1143) projected
  line L448 (-133, -24.1143) -> (-133, -18.9143) projected
  line L449 (-129.5, -55.2) -> (-129.5, -54.9) projected
  line L450 (-129.5, -54.9) -> (-127.6, -54.9) projected
  line L451 (-127.6, -54.9) -> (-127.6, -54.2) projected
  line L452 (-127.6, -54.2) -> (-127.3, -54.2) projected
  line L453 (-127.3, -54.2) -> (-127.3, -55.2) projected
  line L454 (-127.3, -55.2) -> (-129.5, -55.2) projected
  line L455 (-138.3, -57.2) -> (-138.3, -52) projected
  line L456 (-138.3, -52) -> (-135.7, -52) projected
  line L457 (-135.7, -52) -> (-135.7, -57.2) projected
  line L458 (-135.7, -57.2) -> (-138.3, -57.2) projected
  line L459 (-128.7, -41.6571) -> (-126, -41.6571) projected
  line L460 (-126, -41.6571) -> (-126, -39.2571) projected
  line L461 (-126, -39.2571) -> (-124.2, -37.4571) projected
  line L462 (-124.2, -37.4571) -> (-119.5, -37.4571) projected
  line L463 (-119.5, -37.4571) -> (-119.5, -38.5571) projected
  line L464 (-119.5, -38.5571) -> (-123.8858, -38.5571) projected
  line L465 (-123.8858, -38.5571) -> (-124.9, -39.5714) projected
  line L466 (-124.9, -39.5714) -> (-124.9, -43.3429) projected
  line L467 (-124.9, -43.3429) -> (-123.8858, -44.3571) projected
  line L468 (-123.8858, -44.3571) -> (-119.5, -44.3571) projected
  line L469 (-119.5, -44.3571) -> (-119.5, -45.4571) projected
  line L470 (-119.5, -45.4571) -> (-124.2, -45.4571) projected
  line L471 (-124.2, -45.4571) -> (-126, -43.6571) projected
  line L472 (-126, -43.6571) -> (-126, -48.3571) projected
  line L473 (-126, -48.3571) -> (-128.7, -48.3571) projected
  line L474 (-128.7, -48.3571) -> (-128.7, -41.6571) projected
  line L475 (-133, -35.4571) -> (-130.7, -35.4571) projected
  line L476 (-130.7, -35.4571) -> (-130.7, -40.6571) projected
  line L477 (-130.7, -40.6571) -> (-133, -40.6571) projected
  line L478 (-133, -40.6571) -> (-133, -35.4571) projected
  line L479 (-129.5, -22.1143) -> (-129.5, -21.8143) projected
  line L480 (-129.5, -21.8143) -> (-127.6, -21.8143) projected
  line L481 (-127.6, -21.8143) -> (-127.6, -21.1143) projected
  line L482 (-127.6, -21.1143) -> (-127.3, -21.1143) projected
  line L483 (-127.3, -21.1143) -> (-127.3, -22.1143) projected
  line L484 (-127.3, -22.1143) -> (-129.5, -22.1143) projected
  line L485 (-129.5, -5.5714) -> (-129.5, -5.2714) projected
  line L486 (-129.5, -5.2714) -> (-127.6, -5.2714) projected
  line L487 (-127.6, -5.2714) -> (-127.6, -4.5714) projected
  line L488 (-127.6, -4.5714) -> (-127.3, -4.5714) projected
  line L489 (-127.3, -4.5714) -> (-127.3, -5.5714) projected
  line L490 (-127.3, -5.5714) -> (-129.5, -5.5714) projected
  line L491 (-138.3, -7.5714) -> (-138.3, -2.3714) projected
  line L492 (-138.3, -2.3714) -> (-135.7, -2.3714) projected
  line L493 (-135.7, -2.3714) -> (-135.7, -7.5714) projected
  line L494 (-135.7, -7.5714) -> (-138.3, -7.5714) projected
  line L495 (-138.3, 25.5143) -> (-138.3, 30.7143) projected
  line L496 (-138.3, 30.7143) -> (-135.7, 30.7143) projected
  line L497 (-135.7, 30.7143) -> (-135.7, 25.5143) projected
  line L498 (-135.7, 25.5143) -> (-138.3, 25.5143) projected
  line L499 (-128.7, 57.6) -> (-126, 57.6) projected
  line L500 (-126, 57.6) -> (-126, 60) projected
  line L501 (-126, 60) -> (-124.2, 61.8) projected
  line L502 (-124.2, 61.8) -> (-119.5, 61.8) projected
  line L503 (-119.5, 61.8) -> (-119.5, 60.7) projected
  line L504 (-119.5, 60.7) -> (-123.8858, 60.7) projected
  line L505 (-123.8858, 60.7) -> (-124.9, 59.6858) projected
  line L506 (-124.9, 59.6858) -> (-124.9, 55.9142) projected
  line L507 (-124.9, 55.9142) -> (-123.8858, 54.9) projected
  line L508 (-123.8858, 54.9) -> (-119.5, 54.9) projected
  line L509 (-119.5, 54.9) -> (-119.5, 53.8) projected
  line L510 (-119.5, 53.8) -> (-124.2, 53.8) projected
  line L511 (-124.2, 53.8) -> (-126, 55.6) projected
  line L512 (-126, 55.6) -> (-126, 50.9) projected
  line L513 (-126, 50.9) -> (-128.7, 50.9) projected
  line L514 (-128.7, 50.9) -> (-128.7, 57.6) projected
  line L515 (-133, 58.6) -> (-133, 63.8) projected
  line L516 (-133, 63.8) -> (-130.7, 63.8) projected
  line L517 (-130.7, 63.8) -> (-130.7, 58.6) projected
  line L518 (-130.7, 58.6) -> (-133, 58.6) projected
  line L519 (-127.3, 45.0571) -> (-127.3, 44.0571) projected
  line L520 (-127.3, 44.0571) -> (-129.5, 44.0571) projected
  line L521 (-129.5, 44.0571) -> (-129.5, 44.3571) projected
  line L522 (-129.5, 44.3571) -> (-127.6, 44.3571) projected
  line L523 (-127.6, 44.3571) -> (-127.6, 45.0571) projected
  line L524 (-127.6, 45.0571) -> (-127.3, 45.0571) projected
  line L525 (-129.5, 27.5143) -> (-129.5, 27.8143) projected
  line L526 (-129.5, 27.8143) -> (-127.6, 27.8143) projected
  line L527 (-127.6, 27.8143) -> (-127.6, 28.5143) projected
  line L528 (-127.6, 28.5143) -> (-127.3, 28.5143) projected
  line L529 (-127.3, 28.5143) -> (-127.3, 27.5143) projected
  line L530 (-127.3, 27.5143) -> (-129.5, 27.5143) projected
  line L531 (-135.5, 30.7143) -> (-133.2, 30.7143) projected
  line L532 (-133.2, 30.7143) -> (-133.2, 25.5143) projected
  line L533 (-133.2, 25.5143) -> (-135.5, 25.5143) projected
  line L534 (-135.5, 25.5143) -> (-135.5, 30.7143) projected
  line L535 (-127.3, -2.3714) -> (-127.3, -3.3714) projected
  line L536 (-127.3, -3.3714) -> (-127.6, -3.3714) projected
  line L537 (-127.6, -3.3714) -> (-127.6, -2.6714) projected
  line L538 (-127.6, -2.6714) -> (-129.5, -2.6714) projected
  line L539 (-129.5, -2.6714) -> (-129.5, -2.3714) projected
  line L540 (-129.5, -2.3714) -> (-127.3, -2.3714) projected
  line L541 (-127.3, -18.9143) -> (-127.3, -19.9143) projected
  line L542 (-127.3, -19.9143) -> (-127.6, -19.9143) projected
  line L543 (-127.6, -19.9143) -> (-127.6, -19.2143) projected
  line L544 (-127.6, -19.2143) -> (-129.5, -19.2143) projected
  line L545 (-129.5, -19.2143) -> (-129.5, -18.9143) projected
  line L546 (-129.5, -18.9143) -> (-127.3, -18.9143) projected
  line L547 (-137, -31.8143) -> (-137, -26.2143) projected
  line L548 (-137, -26.2143) -> (-131, -26.2143) projected
  line L549 (-131, -26.2143) -> (-131, -31.8143) projected
  line L550 (-131, -31.8143) -> (-137, -31.8143) projected
  line L551 (-128.7, -58.2) -> (-126, -58.2) projected
  line L552 (-126, -58.2) -> (-126, -55.8) projected
  line L553 (-126, -55.8) -> (-124.2, -54) projected
  line L554 (-124.2, -54) -> (-119.5, -54) projected
  line L555 (-119.5, -54) -> (-119.5, -55.1) projected
  line L556 (-119.5, -55.1) -> (-123.8858, -55.1) projected
  line L557 (-123.8858, -55.1) -> (-124.9, -56.1142) projected
  line L558 (-124.9, -56.1142) -> (-124.9, -59.8858) projected
  line L559 (-124.9, -59.8858) -> (-123.8858, -60.9) projected
  line L560 (-123.8858, -60.9) -> (-119.5, -60.9) projected
  line L561 (-119.5, -60.9) -> (-119.5, -62) projected
  line L562 (-119.5, -62) -> (-124.2, -62) projected
  line L563 (-124.2, -62) -> (-126, -60.2) projected
  line L564 (-126, -60.2) -> (-126, -64.9) projected
  line L565 (-126, -64.9) -> (-128.7, -64.9) projected
  line L566 (-128.7, -64.9) -> (-128.7, -58.2) projected
  line L567 (-137, -64.9) -> (-137, -59.3) projected
  line L568 (-137, -59.3) -> (-131, -59.3) projected
  line L569 (-131, -59.3) -> (-131, -64.9) projected
  line L570 (-131, -64.9) -> (-137, -64.9) projected
  circle A135 centre (50, 13.375) radius 1.5 projected
  circle A136 centre (50, -44.625) radius 1.5 projected
  circle A137 centre (76.5, 13.375) radius 1.5 projected
  circle A138 centre (76.5, -44.625) radius 1.5 projected
  line L571 (82, 17.75) -> (82, -49) projected
  line L572 (44.5, 17.75) -> (82, 17.75) projected
  line L573 (44.5, -49) -> (44.5, 17.75) projected
  line L574 (82, -49) -> (44.5, -49) projected
  line L575 (64.75, 67.25) -> (65.25, 67.75) projected
  line L576 (65.25, 67.75) -> (66.75, 67.75) projected
  line L577 (66.75, 67.75) -> (67.25, 67.25) projected
  line L578 (67.25, 67.25) -> (67.25, 65.75) projected
  line L579 (67.25, 65.75) -> (66.75, 65.25) projected
  line L580 (66.75, 65.25) -> (65.25, 65.25) projected
  line L581 (65.25, 65.25) -> (64.75, 65.75) projected
  line L582 (64.75, 65.75) -> (64.25, 65.25) projected
  line L583 (64.25, 65.25) -> (62.75, 65.25) projected
  line L584 (62.75, 65.25) -> (62.25, 65.75) projected
  line L585 (62.25, 65.75) -> (61.75, 65.25) projected
  line L586 (61.75, 65.25) -> (60.25, 65.25) projected
  line L587 (60.25, 65.25) -> (59.75, 65.75) projected
  line L588 (59.75, 65.75) -> (59.75, 67.25) projected
  line L589 (59.75, 67.25) -> (60.25, 67.75) projected
  line L590 (60.25, 67.75) -> (61.75, 67.75) projected
  line L591 (61.75, 67.75) -> (62.25, 67.25) projected
  line L592 (62.25, 67.25) -> (62.75, 67.75) projected
  line L593 (62.75, 67.75) -> (64.25, 67.75) projected
  line L594 (64.25, 67.75) -> (64.75, 67.25) projected
  circle A139 centre (53.5, 69.25) radius 1.6 projected
  circle A140 centre (73.5, 69.25) radius 1.6 projected
  line L595 (48.5, 71.75) -> (48.5, 27.75) projected
  line L596 (48.5, 27.75) -> (78.5, 27.75) projected
  line L597 (78.5, 27.75) -> (78.5, 71.75) projected
  line L598 (78.5, 71.75) -> (76.5, 73.75) projected
  line L599 (76.5, 73.75) -> (50.5, 73.75) projected
  line L600 (50.5, 73.75) -> (48.5, 71.75) projected
  line L601 (62.6, 33.15) -> (54.4, 33.15) projected
  line L602 (54.4, 33.15) -> (54.4, 31.75) projected
  line L603 (54.4, 31.75) -> (52.6, 31.75) projected
  line L604 (52.6, 31.75) -> (52.6, 46.55) projected
  line L605 (52.6, 46.55) -> (54.4, 46.55) projected
  line L606 (54.4, 46.55) -> (54.4, 45.15) projected
  line L607 (54.4, 45.15) -> (62.6, 45.15) projected
  line L608 (62.6, 45.15) -> (62.6, 46.55) projected
  line L609 (62.6, 46.55) -> (64.4, 46.55) projected
  line L610 (64.4, 46.55) -> (64.4, 45.15) projected
  line L611 (64.4, 45.15) -> (72.6, 45.15) projected
  line L612 (72.6, 45.15) -> (72.6, 46.55) projected
  line L613 (72.6, 46.55) -> (74.4, 46.55) projected
  line L614 (74.4, 46.55) -> (74.4, 31.75) projected
  line L615 (74.4, 31.75) -> (72.6, 31.75) projected
  line L616 (72.6, 31.75) -> (72.6, 33.15) projected
  line L617 (72.6, 33.15) -> (64.4, 33.15) projected
  line L618 (64.4, 33.15) -> (64.4, 31.75) projected
  line L619 (64.4, 31.75) -> (62.6, 31.75) projected
  line L620 (62.6, 31.75) -> (62.6, 33.15) projected
  circle A141 centre (155.5, 44.5) radius 1.5 projected
  circle A142 centre (155.5, -40.5) radius 1.5 projected
  circle A143 centre (155.5, -40.5) radius 1.5 projected
  point P0 (0, 0)
hole "Hole1" at (-195.4, 74.75, 6) at (-195.4, 34.75, 6) at (-155.4, 34.75, 6) at (-155.4, 74.75, 6) at (-195.4, 20.25, 6) at (-155.4, 20.25, 6) at (-155.4, -19.75, 6) at (-195.4, -19.75, 6) at (-195.4, -34.25, 6) at (-155.4, -34.25, 6) at (-155.4, -74.25, 6) at (-195.4, -74.25, 6) at (-141, -66, 6) at (-97, -66, 6) at (-97, 66, 6) at (-141, 66, 6) at (53.5, 69.25, 6) at (73.5, 69.25, 6) at (76.5, 13.375, 6) at (50, 13.375, 6) at (76.5, -44.625, 6) at (50, -44.625, 6) at (155.5, -40.5, 6) at (155.5, 44.5, 6) direction (0, 0, -1) diameter 2 depth 6 tip angle 90
sketch "Sketch4" plane through (0, 0, 6) normal (0, 0, 1) x (1, 0, 0)
  line L0 (123.5293, 57.7) -> (117.4707, 57.7) projected
  line L1 (117.4707, 57.7) -> (123.5293, 57.7) projected
  line L2 (122.37, 57.7) -> (118.63, 57.7) projected
  line L3 (135, 94) -> (105, 94) projected
  line L4 (117.2707, 65.85) -> (111.2707, 65.85)
  line L5 (111.2707, 65.85) -> (111.2707, 85.85)
  line L6 (111.2707, 85.85) -> (117.2707, 85.85)
  line L7 (117.2707, 85.85) -> (117.2707, 65.85)
  line L8 (123.7293, 65.85) -> (129.7293, 65.85)
  line L9 (129.7293, 65.85) -> (129.7293, 85.85)
  line L10 (129.7293, 85.85) -> (123.7293, 85.85)
  line L11 (123.7293, 85.85) -> (123.7293, 65.85)
  line L12 (117.4707, 57.7) -> (117.4707, 94) construction
  line L13 (123.5293, 57.7) -> (123.5293, 94) construction
  point P0 (0, 0)
  point P1 (117.2707, 75.85)
  point P2 (117.4707, 75.85)
  dimension "d46" = 0.2
  dimension "d47" = 0.2
  dimension "d48" = 6
  dimension "d49" = 20
  constraints: 20 end point, 4 parallel, 4 perpendicular, 4 point on line, 2 horizontal, 2 midpoint, 1 collinear, 1 horizontal alignment
  measures "d46" distance between parallel lines of L12 L7
  measures "d47" distance between parallel lines of L11 L13
  measures "d48" distance of L8.start L8.end
  measures "d49" distance of L4.end L5.end
extrude "Cut2" cut sketch "Sketch4" against normal blind 6
equation "\"d12\" = d2"
equation "\"d15\" = d13"
equation "\"d30\" = d29"
equation "\"d32\" = d31"
equation "\"d37\" = Thickness"
equation "\"d44\" = Thickness"
equation "\"d47\" = d46"
equation "\"d50\" = Thickness"
equation "\"d33\" = Thickness"
equation "\"BendRadius\" = Thickness"
equation "\"BendReliefWidth\" = Thickness"
equation "\"BendReliefDepth\" = 0.5 * Thickness"
equation "\"CornerReliefSize\" = 4 * Thickness"
equation "\"MinimumRemnant\" = 2 * Thickness"
equation "\"TransitionRadius\" = BendRadius"
equation "\"JacobiRadiusSize\" = BendRadius"
equation "\"GapSize\" = Thickness"
equation "\"Thickness\" = 6"
body "Solid1"
